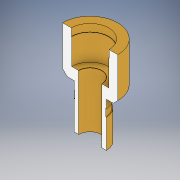
# Autodesk Inventor part: fridge bushing
Saved by Autodesk Inventor 2018 (Build 220112000, 112)
## iProperties
Created: 2019-03-26
Part Number: fridge bushing
Material: Brass
Document SubType Name: Modeling
Designer: Admin
Density: 8.49 g/cm^3
Appearance: Brass - Polished
Author: Admin
Autodesk Inventor part; units mm, degrees
ref_plane "YZ Plane" through (0, 0, 0) normal (1, 0, 0) x (0, 1, 0)
ref_plane "XZ Plane" through (0, 0, 0) normal (0, 1, 0) x (-1, 0, 0)
ref_plane "XY Plane" through (0, 0, 0) normal (0, 0, 1) x (1, 0, 0)
sketch "Sketch1" plane through (0, 0, 0) normal (0, 1, 0) x (-1, 0, 0)
  circle A0 centre (0, 0) radius 9.525
  dimension "d0" = 19.05
  constraints: 1 centre point, 1 coincident
  measures "d0" diameter of A0
extrude "Extrusion1" add sketch "Sketch1" along normal mid plane 30.48
sketch "Sketch3" plane through (0, 15.24, 0) normal (0, 1, 0) x (1, 0, 0)
  point P0 (0, 0)
  point P1 (0, 0)
  constraints: 1 coincident
hole "Hole1" at (0, 15.24, 0) direction (0, -1, 0) diameter 7.9375 end through all
sketch "Sketch4" plane through (0, 15.24, 0) normal (0, 1, 0) x (1, 0, 0)
  point P0 (0, 0)
  point P1 (0, 0)
  constraints: 1 coincident
hole "Hole2" at (0, 15.24, 0) direction (0, -1, 0) diameter 12.3031 depth 10.16 tip angle 118
sketch "Sketch5" plane through (0, 15.24, 0) normal (0, 1, 0) x (1, 0, 0)
  circle A0 centre (0, 0) radius 6.3627
  dimension "d20" = 12.7254
  constraints: 1 centre point, 1 coincident
  measures "d20" diameter of A0
extrude "Extrusion3" cut sketch "Sketch5" against normal blind 11.43
sketch "Sketch6" plane through (0, 15.24, 0) normal (0, 1, 0) x (1, 0, 0)
  circle A0 centre (0, 0) radius 6.477
  dimension "d23" = 12.954
  constraints: 1 centre point, 1 coincident
  measures "d23" diameter of A0
extrude "Extrusion4" cut sketch "Sketch6" against normal blind 2.54
sketch "Sketch7" plane through (0, -15.24, 0) normal (0, -1, 0) x (1, 0, 0)
  circle A0 centre (0, 0) radius 9.525
  circle A1 centre (0, 0) radius 9.525 projected
  circle A2 centre (0, 0) radius 5.5753
  dimension "d26" = 11.1506
  constraints: 2 centre point, 2 coincident, 1 concentric
  measures "d26" diameter of A2
extrude "Extrusion5" cut sketch "Sketch7" against normal blind 15.24
sketch "Sketch9" plane through (0, 0, 0) normal (0, 0, 1) x (1, 0, 0)
  line L0 (3.9688, -15.24) -> (-3.9688, -15.24) projected
  line L1 (0, -15.24) -> (0, -4.064) construction
  line L2 (0, -15.24) -> (11.176, -15.24) construction
  line L3 (0, -4.064) -> (5.461, -4.064) construction
  line L4 (5.5753, -15.24) -> (5.5753, 0) projected
  line L5 (5.588, -2.794) -> (5.334, -2.794)
  line L6 (5.334, -2.794) -> (5.334, -5.334)
  line L7 (5.334, -5.334) -> (5.588, -5.334)
  line L8 (5.588, -5.334) -> (5.588, -2.794)
  line L9 (5.588, -2.794) -> (5.334, -5.334) construction
  line L10 (5.334, -2.794) -> (5.588, -5.334) construction
  point P0 (0, 0)
  dimension "d35" = 11.176
  dimension "d36" = 90
  dimension "d37" = 5.461
  dimension "d38" = 90
  dimension "d39" = 0.254
  dimension "d40" = 2.54
  constraints: 18 end point, 3 midpoint, 3 perpendicular, 2 horizontal, 2 parallel, 1 vertical
  measures "d35" distance of L1.start L1.end
  measures "d36" angle of L2 L1
  measures "d37" distance of L1.end L3.end
  measures "d38" angle of L1 L3
  measures "d39" distance of L7.end L6.end
  measures "d40" distance of L6.end L5.end
revolve "Revolution1" cut sketch "Sketch9" angle 360 about axis through (0, -15.24, 0) along (0, 1, 0)
chamfer "Chamfer2" distance 1.5875 angle 45 1 edges at (9.525, 0, 0)
body "Solid1"
